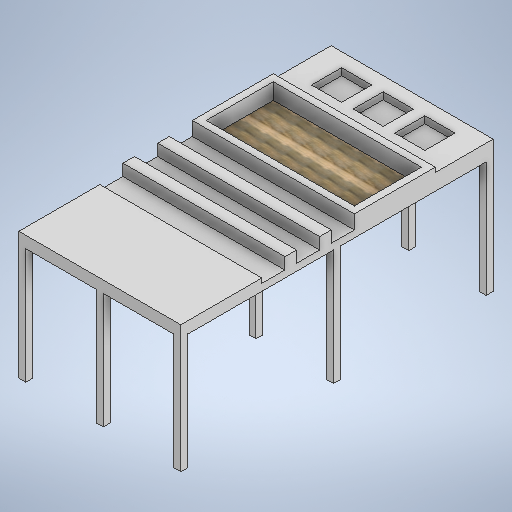
# Autodesk Inventor part: Table
Saved by Autodesk Inventor 2025 (Build 290162000, 162)
## iProperties
Created: 2024-06-19
Part Number: Table
Material: Generic
Document SubType Name: Modeling
Designer: User
Density: 1 g/cm^3
Appearance: Default
Author: User
Autodesk Inventor part; units mm, degrees
ref_plane "YZ Plane" through (0, 0, 0) normal (1, 0, 0) x (0, 1, 0)
ref_plane "XZ Plane" through (0, 0, 0) normal (0, 1, 0) x (-1, 0, 0)
ref_plane "XY Plane" through (0, 0, 0) normal (0, 0, 1) x (1, 0, 0)
sketch "Sketch1" plane through (0, 0, 0) normal (0, 1, 0) x (-1, 0, 0)
  line L0 (-350, 675) -> (350, 675)
  line L1 (350, 675) -> (350, -675)
  line L2 (350, -675) -> (-350, -675)
  line L3 (-350, -675) -> (-350, 675)
  line L4 (-350, 675) -> (350, -675) construction
  line L5 (350, 675) -> (-350, -675) construction
  line L6 (350, 675) -> (-350, 675)
  line L7 (-350, 675) -> (-350, 325)
  line L8 (-350, 325) -> (350, 325)
  line L9 (350, 325) -> (350, 675)
  line L10 (350, 325) -> (-350, 325)
  line L11 (-350, 325) -> (-350, -75)
  line L12 (-350, -75) -> (350, -75)
  line L13 (350, -75) -> (350, 325)
  line L14 (350, -75) -> (-350, -75)
  line L15 (-350, -75) -> (-350, -425)
  line L16 (-350, -425) -> (350, -425)
  line L17 (350, -425) -> (350, -75)
  line L18 (350, -425) -> (-350, -425)
  line L19 (-350, -425) -> (-350, -675)
  line L20 (-350, -675) -> (350, -675)
  line L21 (350, -675) -> (350, -425)
  point P0 (0, 0)
  dimension "d1" = 1350
  dimension "d2" = 700
  dimension "d3" = 350
  dimension "d4" = 400
  dimension "d5" = 350
  constraints: 44 end point, 10 parallel, 5 horizontal, 5 perpendicular, 3 point on line, 2 midpoint
  measures "d1" distance of L0.end L1.end
  measures "d2" distance of L1.end L2.end
  measures "d3" distance of L8.end L0.end
  measures "d4" distance between parallel lines of L12 L8
  measures "d5" distance between parallel lines of L16 L12
extrude "Extrusion1" add sketch "Sketch1" along normal blind 50 contours L0 L1 L8 L3
extrude "Extrusion2" add sketch "Sketch1" along normal blind 30 contours L8 L1 L12 L3
extrude "Extrusion3" add sketch "Sketch1" along normal blind 90 contours L12 L1 L16 L3
extrude "Extrusion4" add sketch "Sketch1" along normal blind 70 contours L16 L1 L2 L3
sketch "Sketch2" plane through (0, 90, 0) normal (0, 1, 0) x (1, 0, 0)
  line L0 (-320, 105) -> (320, 105)
  line L1 (320, 105) -> (320, 395)
  line L2 (320, 395) -> (-320, 395)
  line L3 (-320, 395) -> (-320, 105)
  line L4 (-350, 75) -> (350, 75) projected
  line L5 (-350, 425) -> (-350, 75) projected
  line L6 (350, 75) -> (350, 425) projected
  line L7 (350, 425) -> (-350, 425) projected
  line L8 (-245, 485) -> (-115, 485)
  line L9 (-115, 485) -> (-115, 615)
  line L10 (-115, 615) -> (-245, 615)
  line L11 (-245, 615) -> (-245, 485)
  line L12 (-65, 485) -> (65, 485)
  line L13 (65, 485) -> (65, 615)
  line L14 (65, 615) -> (-65, 615)
  line L15 (-65, 615) -> (-65, 485)
  line L16 (115, 485) -> (245, 485)
  line L17 (245, 485) -> (245, 615)
  line L18 (245, 615) -> (115, 615)
  line L19 (115, 615) -> (115, 485)
  line L20 (-350, 675) -> (-350, 425) projected
  point P0 (0, 0)
  point P1 (320, 250)
  dimension "d14" = 30
  dimension "d15" = 30
  dimension "d16" = 30
  dimension "d17" = 30
  dimension "d18" = 130
  dimension "d19" = 130
  dimension "d20" = 105
  dimension "d21" = 60
  dimension "d22" = 50
  dimension "d23" = 50
  constraints: 32 end point, 8 parallel, 4 equal length, 4 horizontal, 4 perpendicular, 2 point on line, 1 midpoint
  measures "d14" distance between parallel lines of L4 L0
  measures "d15" distance between parallel lines of L5 L3
  measures "d16" distance from line of L6 point (320, 250)
  measures "d17" distance between parallel lines of L7 L2
  measures "d18" distance of L10.end L8.start
  measures "d19" distance of L9.end L10.end
  measures "d20" distance between parallel lines of L20 L11
  measures "d21" distance between parallel lines of L7 L8
  measures "d22" distance between parallel lines of L13 L19
  measures "d23" distance between parallel lines of L9 L15
extrude "Extrusion5" cut sketch "Sketch2" against normal blind 70 contours L3 L2 L1 L0
extrude "Extrusion6" cut sketch "Sketch2" against normal blind 50 contours L11 L10 L9 L8 | L15 L14 L13 L12 | L19 L18 L17 L16
sketch "Sketch4" plane through (0, 0, 0) normal (0, -1, 0) x (1, 0, 0)
  line L0 (-350, -675) -> (-350, 675) projected
  line L1 (-350, 675) -> (-320, 675)
  line L2 (-320, 675) -> (-320, 645)
  line L3 (-320, 645) -> (-350, 645)
  line L4 (-350, 645) -> (-350, 675)
  line L5 (-350, 675) -> (350, 675) projected
  line L6 (350, 675) -> (350, -675) projected
  line L7 (320, 675) -> (350, 675)
  line L8 (350, 675) -> (350, 645)
  line L9 (350, 645) -> (320, 645)
  line L10 (320, 645) -> (320, 675)
  line L11 (-350, -675) -> (-350, -425) projected
  line L12 (-350, -675) -> (-320, -675)
  line L13 (-320, -675) -> (-320, -645)
  line L14 (-320, -645) -> (-350, -645)
  line L15 (-350, -645) -> (-350, -675)
  line L16 (350, -675) -> (320, -675)
  line L17 (320, -675) -> (320, -645)
  line L18 (320, -645) -> (350, -645)
  line L19 (350, -645) -> (350, -675)
  line L20 (-15, 675) -> (15, 675)
  line L21 (15, 675) -> (15, 645)
  line L22 (15, 645) -> (-15, 645)
  line L23 (-15, 645) -> (-15, 675)
  line L24 (350, -675) -> (-350, -675) projected
  line L25 (-15, -675) -> (15, -675)
  line L26 (15, -675) -> (15, -645)
  line L27 (15, -645) -> (-15, -645)
  line L28 (-15, -645) -> (-15, -675)
  line L29 (-350, 15) -> (-320, 15)
  line L30 (-320, 15) -> (-320, -15)
  line L31 (-320, -15) -> (-350, -15)
  line L32 (-350, -15) -> (-350, 15)
  line L33 (320, 15) -> (350, 15)
  line L34 (350, 15) -> (350, -15)
  line L35 (350, -15) -> (320, -15)
  line L36 (320, -15) -> (320, 15)
  line L37 (-15, 15) -> (15, 15)
  line L38 (15, 15) -> (15, -15)
  line L39 (15, -15) -> (-15, -15)
  line L40 (-15, -15) -> (-15, 15)
  point P0 (0, 0)
  point P1 (0, -645)
  point P2 (0, -675)
  point P3 (0, 645)
  point P4 (320, 0)
  point P5 (-320, 0)
  point P6 (-350, 0)
  point P7 (350, 0)
  point P8 (0, 15)
  point P9 (15, 0)
  dimension "d32" = 30
  dimension "d33" = 30
  constraints: 72 end point, 18 parallel, 13 equal length, 11 midpoint, 9 horizontal, 9 perpendicular, 9 point on line, 3 horizontal alignment, 3 vertical alignment
  measures "d32" distance of L1.end L2.end
  measures "d33" distance of L2.end L3.end
extrude "Extrusion8" add sketch "Sketch4" along normal blind 500 contours L0 L14 L13 L12 | L28 L27 L26 L24 | L0 L29 L30 L31 | L17 L18 L6 L16 | L0 L1 L2 L3 | L35 L36 L33 L6 | L5 L21 L22 L23 | L9 L10 L5 L6 | L37 L38 L39 L40
sketch "Sketch5" plane through (0, 30, 0) normal (0, 1, 0) x (1, 0, 0)
  line L0 (-350, 75) -> (-350, -325) projected
  line L1 (350, -325) -> (350, 75) projected
  line L2 (-350, -25) -> (350, -25)
  line L3 (350, -25) -> (350, -75)
  line L4 (350, -75) -> (-350, -75)
  line L5 (-350, -75) -> (-350, -25)
  line L6 (-350, -175) -> (350, -175)
  line L7 (350, -175) -> (350, -225)
  line L8 (350, -225) -> (-350, -225)
  line L9 (-350, -225) -> (-350, -175)
  line L10 (350, -325) -> (-350, -325) projected
  line L11 (-350, 75) -> (350, 75) projected
  point P0 (0, 0)
  point P1 (350, -25)
  point P2 (-350, -225)
  point P3 (350, -175)
  dimension "d36" = 700
  dimension "d37" = 50
  dimension "d38" = 50
  dimension "d39" = 100
  dimension "d40" = 100
  constraints: 16 end point, 4 parallel, 4 point on line, 2 horizontal, 2 perpendicular
  measures "d36" distance of L6.start L6.end
  measures "d37" distance between parallel lines of L4 L2
  measures "d38" distance between parallel lines of L8 L6
  measures "d39" distance between parallel lines of L10 L8
  measures "d40" distance between parallel lines of L11 L2
extrude "Extrusion9" add sketch "Sketch5" along normal blind 50 contours L2 L1 L4 L0 | L6 L1 L8 L0
body "Solid1"
